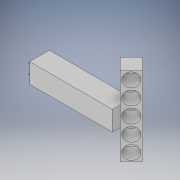
# Autodesk Inventor part: TubeHolderV3
Saved by Autodesk Inventor 2019 (Build 230136000, 136)
## iProperties
Created: 2021-09-16
Part Number: TubeHolderV3
Material: Generic
Document SubType Name: Modeling
Designer: timmy
Density: 1 g/cm^3
Appearance: Default
Author: timmy
Autodesk Inventor part; units mm, degrees
ref_plane "YZ Plane" through (0, 0, 0) normal (1, 0, 0) x (0, 1, 0)
ref_plane "XZ Plane" through (0, 0, 0) normal (0, 1, 0) x (-1, 0, 0)
ref_plane "XY Plane" through (0, 0, 0) normal (0, 0, 1) x (1, 0, 0)
sketch "Sketch1" plane through (0, 0, 0) normal (0, 1, 0) x (-1, 0, 0)
  line L0 (0, 0) -> (0, -50.8)
  line L1 (0, -50.8) -> (76.2, -127)
  line L2 (127, -127) -> (76.2, -127)
  line L3 (0, 0) -> (127, 0)
  line L4 (127, 0) -> (533.4, 0)
  line L5 (533.4, 0) -> (533.4, -127)
  line L6 (533.4, -127) -> (127, -127)
  dimension "d7" = 135
  dimension "d37" = 406.4
  constraints: 14 end point, 3 horizontal, 2 perpendicular
  measures "d7" angle of L1 L0
  measures "d37" distance of L3.end L4.end
extrude "Extrusion1" add sketch "Sketch1" along normal blind 127
sketch "Sketch2" plane through (-76.2, 0, -127) normal (0.7071, 0, -0.7071) x (-0.7071, 0, -0.7071)
  line L0 (-107.7631, 0) -> (0, 0) projected
  line L1 (0, 0) -> (0, 127) projected
  line L2 (-107.7631, 127) -> (0, 127) projected
  line L3 (-107.7631, 0) -> (-107.7631, 127)
  line L4 (-107.7631, -190.5) -> (0.0091, -190.5)
  line L5 (0.0091, -190.5) -> (0.0091, 317.5)
  line L6 (0.0091, 317.5) -> (-107.7631, 317.5)
  line L7 (-107.7631, -190.5) -> (-107.7631, 317.5)
  point P0 (-143.6841, 0)
  dimension "d9" = 107.7722
  dimension "d10" = 508
  constraints: 10 end point, 2 perpendicular, 1 horizontal, 1 vertical
  measures "d9" distance of L4.start L4.end
  measures "d10" distance of L4.end L5.end
extrude "Extrusion2" add sketch "Sketch2" along normal blind 101.6
sketch "Sketch3" plane through (-76.2065, -190.5, -127.0065) normal (-0.7071, 0, -0.7071) x (-0.7071, 0, 0.7071)
  line L0 (0, 0) -> (-101.6, 0) projected
  line L1 (0, 508) -> (-101.6, 508) projected
  circle A0 centre (-50.8, 50.8) radius 44.45
  circle A1 centre (-50.8, 152.4) radius 44.45
  circle A2 centre (-50.8, 254) radius 44.45
  circle A3 centre (-50.8, 355.6) radius 44.45
  circle A4 centre (-50.8, 457.2) radius 44.45
  point P0 (35.921, 190.5)
  constraints: 5 centre point
extrude "Extrusion3" cut sketch "Sketch3" against normal blind 127
sketch "Sketch4" plane through (-533.4, 0, -127) normal (-1, 0, 0) x (0, 0, 1)
  line L0 (0, 0) -> (0, 127) construction
  line L1 (76.2, 0) -> (0, 0) construction
  line L2 (0, 63.5) -> (76.2, 0) construction
  line L3 (76.2, 0) -> (127, 63.5) construction
  line L4 (127, 0) -> (127, 127) construction
  line L5 (76.2, 127) -> (0, 127) construction
  line L6 (0, 63.5) -> (76.2, 127) construction
  line L7 (76.2, 127) -> (127, 63.5) construction
  line L8 (38.1, 31.75) -> (101.6, 31.75) construction
  line L9 (38.1, 95.25) -> (101.6, 95.25) construction
  circle A0 centre (38.1, 31.75) radius 6.35
  circle A1 centre (38.1, 95.25) radius 6.35
  circle A2 centre (101.6, 95.25) radius 6.35
  circle A3 centre (101.6, 31.75) radius 6.35
  dimension "d38" = 12.7
  dimension "d39" = 12.7
  dimension "d40" = 12.7
  dimension "d41" = 12.7
  constraints: 12 end point, 6 midpoint, 4 centre point, 4 coincident
  measures "d38" diameter of A0
  measures "d39" diameter of A1
  measures "d40" diameter of A2
  measures "d41" diameter of A3
extrude "Extrusion4" add sketch "Sketch4" along normal blind 25.4
thread "Thread1" size "1/2-13 UNC" class "2A" standard "ANSI Unified Screw Threads" full length
thread "Thread2" size "1/2-13 UNC" class "2A" standard "ANSI Unified Screw Threads" full length
thread "Thread3" size "1/2-13 UNC" class "2A" standard "ANSI Unified Screw Threads" full length
thread "Thread4" size "1/2-13 UNC" class "2A" standard "ANSI Unified Screw Threads" full length
body "Solid1"
